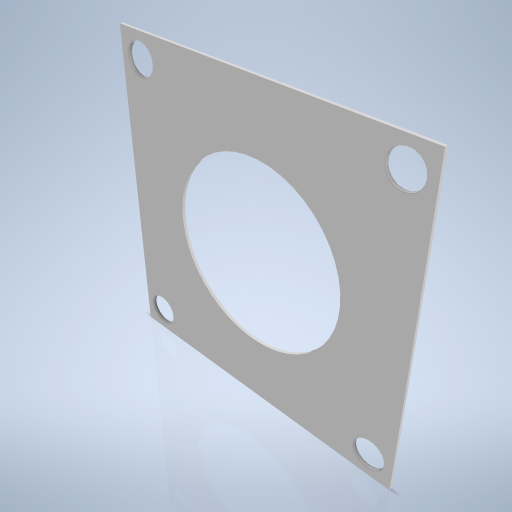
# Autodesk Inventor part: sheet_cylinder
Saved by Autodesk Inventor 2024.2 (Build 282272000, 272)
## iProperties
Created: 2024-05-15
Part Number: sheet_cylinder
Material: Generisch
Document SubType Name: Sheet Metal
Designer: Fabri
Density: 1 g/cm^3
Sheet Metal Rule: Standard_mm
Appearance: Vorgabe
Author: Fabri
Autodesk Inventor part; units mm, degrees
ref_plane "YZ Plane" through (0, 0, 0) normal (1, 0, 0) x (0, 1, 0)
ref_plane "XZ Plane" through (0, 0, 0) normal (0, 1, 0) x (-1, 0, 0)
ref_plane "XY Plane" through (0, 0, 0) normal (0, 0, 1) x (1, 0, 0)
sketch "Skizze1" plane through (0, 0, 0) normal (0, 1, 0) x (-1, 0, 0)
  line L0 (-25, 25) -> (25, 25)
  line L1 (25, 25) -> (25, -25)
  line L2 (25, -25) -> (-25, -25)
  line L3 (-25, -25) -> (-25, 25)
  line L4 (-25, 25) -> (25, -25) construction
  line L5 (25, 25) -> (-25, -25) construction
  point P0 (0, 0)
  dimension "d0" = 50
  dimension "d1" = 50
  measures "d0" distance of L1.end L2.end
  measures "d1" distance of L0.end L1.end
extrude "Grobblech1" add sketch "Skizze1" along normal blind 0.5
sketch "Skizze2" plane through (0, 0.5, 0) normal (0, 1, 0) x (1, 0, 0)
  point P0 (0, 0)
  point P1 (0, 0)
  constraints: 1 coincident
hole "Bohrung1" at (0, 0.5, 0) direction (0, -1, 0) diameter 29 depth 0.5
sketch "Skizze3" plane through (0, 0.5, 0) normal (0, 1, 0) x (1, 0, 0)
  line L0 (-25, -25) -> (25, -25) projected
  line L1 (0, -25) -> (0, 25) construction
  line L2 (25, 25) -> (-25, 25) projected
  line L3 (-25, 25) -> (-25, -25) projected
  line L4 (-25, 0) -> (25.0844, 0) construction
  point P0 (0, 0)
  point P1 (-21.124, -21.124)
  point P2 (-21.124, 21.124)
  point P3 (21.124, -21.124)
  point P4 (21.124, 21.124)
  dimension "d17" = 42.248
  dimension "d19" = 42.248
  constraints: 4 end point, 3 midpoint, 2 horizontal alignment, 2 symmetric about line, 2 vertical alignment, 1 horizontal
  measures "d17" distance of point (21.124, 21.124) point (21.124, -21.124)
  measures "d19" distance of point (21.124, -21.124) point (-21.124, -21.124)
hole "Bohrung2" at (-21.124, 0.5, 21.124) at (-21.124, 0.5, -21.124) at (21.124, 0.5, 21.124) at (21.124, 0.5, -21.124) direction (0, -1, 0) diameter 5 depth 0.5
equation "\"d8\" = Stärke"
equation "\"d2\" = Stärke"
equation "\"Biegeradius\" = Stärke"
equation "\"BreiteBiegungsfreistellung\" = Stärke"
equation "\"TiefeBiegungsfreistellung\" = 0.5 * Stärke"
equation "\"GrößeEckenfreistellung\" = 4 * Stärke"
equation "\"MinimalRest\" = 2 * Stärke"
equation "\"Übergangsradius\" = Biegeradius"
equation "\"JacobiRadiusGröße\" = Biegeradius"
equation "\"Abstandsgröße\" = Stärke"
equation "\"Stärke\" = 0.5"
